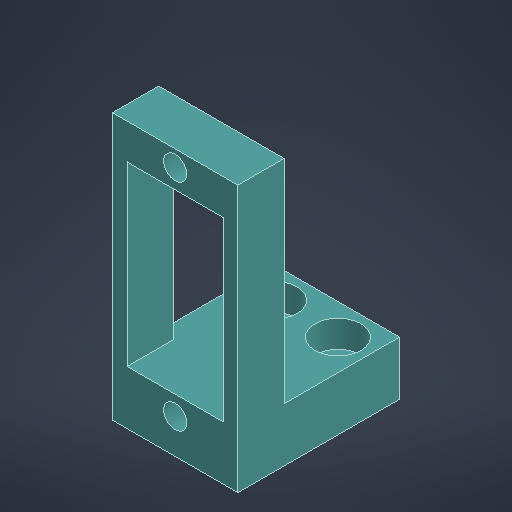
# Autodesk Inventor part: ServoHolder
Saved by Autodesk Inventor 2025.1 (Build 291241000, 241)
## iProperties
Created: 2025-02-09
Part Number: ServoHolder
Material: Generic
Document SubType Name: Modeling
Designer: 13156
Density: 1 g/cm^3
Appearance: Default
Author: 13156
## iProperties of the stored document ServoHolder_3DPrint.ipt
Created: 2025-02-17
Part Number: ServoHolder_3DPrint
Material: Generic
Document SubType Name: Modeling
Designer: jerem
Density: 1 g/cm^3
Appearance: Default
Author: jerem
Autodesk Inventor part; units mm, degrees
ref_plane "YZ Plane" through (0, 0, 0) normal (1, 0, 0) x (0, 1, 0)
ref_plane "XZ Plane" through (0, 0, 0) normal (0, 1, 0) x (-1, 0, 0)
ref_plane "XY Plane" through (0, 0, 0) normal (0, 0, 1) x (1, 0, 0)
sketch "Sketch1" plane through (0, 0, 0) normal (1, 0, 0) x (0, 1, 0)
  line L0 (34.6, 0) -> (0, 0)
  line L1 (0, 0) -> (0, -40)
  line L2 (7, -40) -> (7, -5)
  line L3 (7, -5) -> (34.6, -5)
  line L4 (34.6, -5) -> (34.6, 0)
  line L5 (7, -40) -> (0, -40)
  dimension "d0" = 0
  dimension "d1" = 0
  dimension "d2" = 5
  dimension "d3" = 7
  dimension "d5" = 40
  dimension "d6" = 34.6
  constraints: 12 end point, 3 perpendicular, 2 horizontal, 1 vertical
  measures "d0" distance from line of point (0, 0) L1
  measures "d1" distance from line of point (0, 0) L0
  measures "d2" distance of L3.end L0.start
  measures "d3" distance of L2.start L1.end
  measures "d5" distance of L0.end L1.end
  measures "d6" distance of L0.start L0.end
extrude "Extrusion1" add sketch "Sketch1" along normal blind 16.3
sketch "Sketch2" plane through (0, 7, -5) normal (0, 1, 0) x (1, 0, 0)
  line L0 (16.3, 35) -> (16.3, 0) projected
  line L1 (0, -5) -> (16.3, -5) projected
  circle A0 centre (12.3, 12) radius 1.7
  line L2 (12.3, 5) -> (12.3, 12) construction
  circle A1 centre (4, 12) radius 1.7
  line L3 (0, 35) -> (0, 0) projected
  line L4 (0, 0) -> (16.3, 0) projected
  dimension "d9" = 4
  dimension "d31" = 3.4
  dimension "d46" = 4
  dimension "d47" = 12
  dimension "d48" = 0
  constraints: 2 centre point, 2 end point, 1 equal radius, 1 vertical
  measures "d9" distance from line of L0 L2.start
  measures "d31" diameter of A0
  measures "d46" distance from line of L3 A1.centre
  measures "d47" distance from line of L4 A1.centre
  measures "d48" vertical distance of A1.centre L2.end
extrude "Extrusion2" cut sketch "Sketch2" against normal through all
sketch "Sketch3" plane through (0, 7, -5) normal (0, 0, -1) x (-1, 0, 0)
  line L0 (0, 0) -> (-16.3, 0) projected
  line L1 (-14.4, 0) -> (-1.9, 0)
  line L2 (-1.9, 0) -> (-1.9, 23)
  line L3 (-1.9, 23) -> (-14.4, 23)
  line L4 (-14.4, 23) -> (-14.4, 0)
  line L5 (0, 0) -> (0, 27.6) projected
  point P0 (0, -7)
  dimension "d14" = 23
  dimension "d15" = 12.5
  dimension "d16" = 1.9
  constraints: 8 end point, 2 parallel, 1 horizontal, 1 perpendicular, 1 point on line
  measures "d14" distance of L3.end L1.start
  measures "d15" distance of L2.end L3.end
  measures "d16" distance between parallel lines of L5 L2
extrude "Extrusion3" cut sketch "Sketch3" against normal blind 16.3
sketch "Sketch5" plane through (0, 7, -5) normal (0, 0, -1) x (-1, 0, 0)
  line L0 (0, 27.6) -> (-16.3, 27.6) projected
  line L1 (-16.3, 27.6) -> (0, 27.6)
  line L2 (0, 27.6) -> (0, 0)
  line L3 (0, 0) -> (-1.9, 0)
  line L4 (-14.4, 23) -> (-14.4, 0) projected
  line L5 (-14.4, 23) -> (-14.4, 0)
  line L6 (-14.4, 0) -> (-16.3, 0)
  line L7 (-16.3, 0) -> (-16.3, 27.6)
  line L8 (-14.4, 23) -> (-1.9, 23)
  line L9 (-1.9, 23) -> (-1.9, 0)
  line L10 (-1.9, 23) -> (-1.9, 0) projected
  line L11 (-14.4, 23) -> (-1.9, 23) projected
  point P0 (0, -7)
  dimension "d26" = 0
  dimension "d27" = 0
  dimension "d28" = 1.9
  constraints: 16 end point, 3 perpendicular, 2 horizontal, 1 collinear, 1 parallel, 1 point on line
  measures "d26" distance between parallel lines of L10 L9
  measures "d27" distance between parallel lines of L11 L8
  measures "d28" distance of L4.end L6.end
extrude "Extrusion5" add sketch "Sketch5" along normal blind 4
sketch "Sketch4" plane through (0, 0, 0) normal (0, 0, 1) x (1, 0, 0)
  circle A0 centre (8.15, 32.5) radius 1.5
  circle A1 centre (8.15, 4.5) radius 1.5
  line L0 (1.9, 30) -> (14.4, 30) projected
  line L1 (14.4, 7) -> (1.9, 7) projected
  line L2 (0, 34.6) -> (0, 0) projected
  line L3 (16.3, 34.6) -> (16.3, 0) projected
  dimension "d19" = 2.5
  dimension "d20" = 2.5
  dimension "d21" = 3
  dimension "d22" = 8.15
  dimension "d23" = 8.15
  constraints: 2 centre point, 1 equal radius
  measures "d19" distance from line of L0 A0.centre
  measures "d20" distance from line of L1 A1.centre
  measures "d21" diameter of A1
  measures "d22" distance from line of L2 A0.centre
  measures "d23" distance from line of L3 A1.centre
extrude "Extrusion4" cut sketch "Sketch4" against normal blind 7
sketch "Sketch7" plane through (0, 34.6, 0) normal (0, 1, 0) x (1, 0, 0)
  line L0 (16.3, 0) -> (16.3, 9) projected
  line L1 (0, 0) -> (0, 9) projected
  line L2 (16.3, 9) -> (0, 9)
  line L3 (0, 9) -> (0, 6)
  line L4 (0, 6) -> (16.3, 6)
  line L5 (16.3, 6) -> (16.3, 9)
  line L6 (0, 0) -> (16.3, 0) projected
  dimension "d40" = 6
  constraints: 8 end point, 2 parallel, 1 horizontal, 1 perpendicular, 1 point on line
  measures "d40" distance between parallel lines of L6 L4
extrude "Extrusion7" cut sketch "Sketch7" against normal up to surface (27.6 mm away) contours L4 L1 L2 L0
sketch "Sketch8" plane through (0, 7, -40) normal (0, 1, 0) x (1, 0, 0)
  line L0 (0, 0) -> (16.3, 0) projected
  line L1 (0, 0) -> (0, -34) projected
  line L2 (16.3, 0) -> (0, 0)
  line L3 (0, 0) -> (0, -19)
  line L4 (0, -19) -> (16.3, -19)
  line L5 (16.3, -19) -> (16.3, 0)
  circle A0 centre (12.3, -23) radius 1.7 projected
  point P0 (0, -40)
  dimension "d43" = 4
  constraints: 8 end point, 2 parallel, 1 horizontal, 1 perpendicular, 1 point on line
  measures "d43" distance from line of A0.centre L4
extrude "Extrusion8" cut sketch "Sketch8" against normal blind 10 contours L0 L5 L4 L1
sketch "Sketch9" plane through (1.9, 7, 0) normal (0, 1, 0) x (1, 0, 0)
  circle A0 centre (2.1, 17) radius 1.7 projected
  circle A1 centre (10.4, 17) radius 1.7 projected
  circle A2 centre (2.1, 17) radius 3
  circle A3 centre (10.4, 17) radius 3
  point P0 (-1.9, 0)
  dimension "d49" = 6
  dimension "d50" = 6
  constraints: 2 centre point, 2 coincident
  measures "d49" diameter of A2
  measures "d50" diameter of A3
extrude "Extrusion9" cut sketch "Sketch9" against normal blind 3.5
equation "\"d50\" = d49"
body "Solid1"
